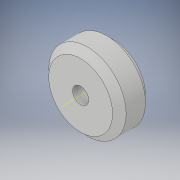
# Autodesk Inventor part: roller
Saved by Autodesk Inventor 2019 (Build 230136000, 136)
## iProperties
Created: 2019-05-06
Part Number: roller
Material: Generic
Document SubType Name: Modeling
Designer: Alex Jones
Density: 1 g/cm^3
Appearance: Default
Author: Alex Jones
Autodesk Inventor part; units mm, degrees
ref_plane "YZ Plane" through (0, 0, 0) normal (1, 0, 0) x (0, 1, 0)
ref_plane "XZ Plane" through (0, 0, 0) normal (0, 1, 0) x (-1, 0, 0)
ref_plane "XY Plane" through (0, 0, 0) normal (0, 0, 1) x (1, 0, 0)
sketch "Sketch2" plane through (0, 0, 0) normal (1, 0, 0) x (0, 1, 0)
  line L0 (12, -3) -> (12, 3)
  line L1 (12, -3) -> (-2.5, 0.625) construction
  line L2 (0, -5.1) -> (9.9, -5.1)
  line L3 (9.9, 5.1) -> (0, 5.1)
  line L4 (9.9, -5.1) -> (-2.5, 1.2879) construction
  line L5 (9.9, 5.1) -> (12, 3)
  line L6 (12, -3) -> (9.9, -5.1)
  line L7 (0, -5.1) -> (2.5, -5.1)
  line L8 (2.5, -5.1) -> (2.5, 5.1)
  line L9 (2.5, 5.1) -> (0, 5.1)
  line L10 (-2.5, -5.1) -> (2.5, 5.1) construction
  line L11 (2.5, -5.1) -> (-2.5, 5.1) construction
  line L12 (-2.5, -0.625) -> (12, 3) construction
  line L13 (-2.5, -1.2879) -> (9.9, 5.1) construction
  line L14 (0, -5.1) -> (0, 5.1)
  point P0 (0, 0)
  dimension "d5" = 6
  dimension "d8" = 10.2
  constraints: 30 end point, 5 point on line, 2 horizontal, 2 midpoint, 2 parallel, 1 perpendicular
  measures "d5" distance of L0.start L0.end
  measures "d8" distance between parallel lines of L2 L3
revolve "Revolution1" add sketch "Sketch2" angle 360 about axis through (0, 0, -5.1) along (0, 0, 1) contours L6 L2 L8 L3 L5 L0
body "Solid1"
